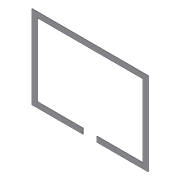
# Autodesk Inventor part: backboardtape
Saved by Autodesk Inventor 2012 (Build 160160000, 160)
## iProperties
Created: 2011-07-01
Part Number: backboardtape
Document SubType Name: Modeling
Designer: dfoster
Density: 1 g/cm^3
Material: Default
Author: dfoster
Autodesk Inventor part; units mm, degrees
ref_plane "YZ Plane" through (0, 0, 0) normal (1, 0, 0) x (0, 1, 0)
ref_plane "XZ Plane" through (0, 0, 0) normal (0, 1, 0) x (-1, 0, 0)
ref_plane "XY Plane" through (0, 0, 0) normal (0, 0, 1) x (1, 0, 0)
sketch "Sketch1" plane through (0, 0, 0) normal (0, 0, 1) x (1, 0, 0)
  line L0 (0, 0) -> (1117.6, 0)
  line L1 (1117.6, 0) -> (1117.6, 800.1)
  line L2 (1117.6, 800.1) -> (0, 800.1)
  line L3 (0, 800.1) -> (0, 0)
  line L4 (50.8, 749.3) -> (1066.8, 749.3)
  line L5 (1066.8, 749.3) -> (1066.8, 50.8)
  line L6 (1066.8, 50.8) -> (50.8, 50.8)
  line L7 (50.8, 50.8) -> (50.8, 749.3)
  dimension "d0" = 800.1
  dimension "d1" = 1117.6
  dimension "d2" = 50.8
  constraints: 16 end point, 4 parallel, 2 perpendicular, 1 horizontal, 3 other
  measures "d0" distance of L2.end L0.start
  measures "d1" distance of L0.start L0.end
  measures "d2" distance between parallel lines of L4 L2
extrude "Extrusion1" add sketch "Sketch1" along normal blind 4.7752
sketch "Sketch2" plane through (0, 0, 4.7752) normal (0, 0, 1) x (1, 0, 0)
  line L0 (1066.8, 50.8) -> (50.8, 50.8) projected
  line L1 (0, 0) -> (0, 800.1) projected
  line L2 (1117.6, 0) -> (0, 0) projected
  line L3 (492.125, 0) -> (625.475, 0)
  line L4 (625.475, 0) -> (625.475, 50.8)
  line L5 (625.475, 50.8) -> (492.125, 50.8)
  line L6 (492.125, 50.8) -> (492.125, 0)
  dimension "d5" = 133.35
  dimension "d6" = 492.125
  constraints: 8 end point, 2 parallel, 2 point on line, 1 horizontal, 1 perpendicular
  measures "d5" distance of L3.start L3.end
  measures "d6" distance between parallel lines of L6 L1
extrude "Extrusion2" cut sketch "Sketch2" against normal through all
body "Solid1"
